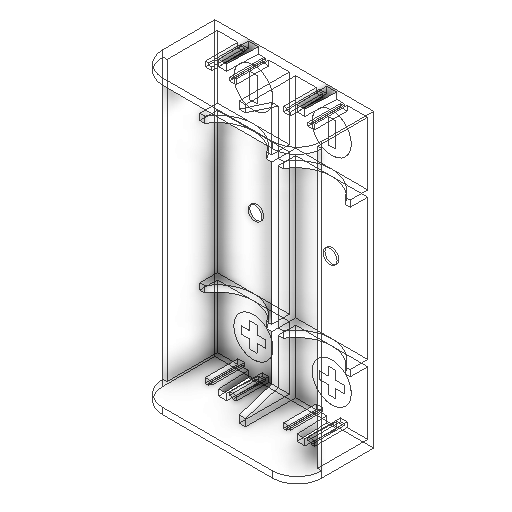
# Autodesk Inventor part: Holder_21700_Dual
Saved by Autodesk Inventor 2025.2 (Build 292293000, 293)
## iProperties
Created: 2025-03-09
Part Number: Holder_21700_Dual
Material: Generic
Document SubType Name: Modeling
Designer: ahorat
Density: 1 g/cm^3
Appearance: Default
Author: ahorat
Autodesk Inventor part; units mm, degrees
ref_plane "YZ Plane" through (0, 0, 0) normal (1, 0, 0) x (0, 1, 0)
ref_plane "XZ Plane" through (0, 0, 0) normal (0, 1, 0) x (-1, 0, 0)
sketch "Sketch1" plane through (0, 0, 0) normal (0, 1, 0) x (-1, 0, 0)
  line L0 (-22.6, 0) -> (22.6, 0)
  line L1 (22.6, 0) -> (22.6, 14.8)
  line L2 (15.6, 21.8) -> (-15.6, 21.8)
  line L3 (-22.6, 14.8) -> (-22.6, 0)
  arc A0 (-15.6, 21.8) -> (-22.6, 14.8) centre (-15.6, 14.8) ccw
  arc A1 (22.6, 14.8) -> (15.6, 21.8) centre (15.6, 14.8) ccw
  point P0 (0, 0)
  point P1 (22.6, 21.8)
  point P2 (0, 0)
  dimension "d0" = 21.8
  dimension "d1" = 45.2
  dimension "d2" = 7
  constraints: 8 end point, 4 point on circle, 4 tangent, 2 centre point, 2 parallel, 2 point on line, 1 coincident, 1 equal radius, 1 horizontal, 1 midpoint, 1 perpendicular
  measures "d0" distance of L0.end point (22.6, 21.8)
  measures "d1" distance between parallel lines of L3 L1
  measures "d2" radius of A0
extrude "Extrusion1" add sketch "Sketch1" along normal mid plane 83
sketch "Sketch2" plane through (-15.6, 41.5, 21.8) normal (0, 0, 1) x (1, 0, 0)
  line L0 (37, -81.2) -> (-5.8, -81.2)
  line L1 (-5.8, -81.2) -> (-5.8, -1.8)
  line L2 (-5.8, -1.8) -> (37, -1.8)
  line L3 (37, -1.8) -> (37, -81.2)
  line L4 (37, -81.2) -> (-5.8, -1.8) construction
  line L5 (-5.8, -81.2) -> (37, -1.8) construction
  line L6 (0, 0) -> (31.2, 0) projected
  line L7 (-7, -83) -> (-7, 0) projected
  point P0 (15.6, -41.5)
  dimension "d5" = 1.8
  dimension "d6" = 1.2
  constraints: 12 end point, 2 midpoint, 2 parallel, 1 horizontal, 1 perpendicular
  measures "d5" distance between parallel lines of L6 L2
  measures "d6" distance between parallel lines of L7 L1
extrude "Extrusion2" cut sketch "Sketch2" against normal blind 21.3
sketch "Sketch3" plane through (-15.6, -41.5, 21.8) normal (0, 0, 1) x (1, 0, 0)
  line L0 (65.6667, 1.8) -> (-34.4667, 1.8)
  line L1 (-34.4667, 1.8) -> (-34.4667, 81.2)
  line L2 (-34.4667, 81.2) -> (65.6667, 81.2)
  line L3 (65.6667, 81.2) -> (65.6667, 1.8)
  line L4 (65.6667, 1.8) -> (-34.4667, 81.2) construction
  line L5 (-34.4667, 1.8) -> (65.6667, 81.2) construction
  line L6 (0, 81.2) -> (31.2, 81.2) projected
  point P0 (15.6, 41.5)
  point P1 (15.6, 81.2)
  constraints: 12 end point, 4 midpoint, 2 parallel, 1 horizontal, 1 perpendicular
extrude "Extrusion3" cut sketch "Sketch3" against normal up to surface (7 mm away)
sketch "Sketch4" plane through (0, 0, 0) normal (1, 0, 0) x (0, 1, 0)
  line L0 (-39.7, 21.8) -> (-39.7, 14.8) projected
  line L1 (-39.7, 14.8) -> (-37.7, 14.8)
  line L2 (-39.7, 14.8) -> (39.7, 14.8) projected
  line L3 (-34.7, 5.5) -> (34.7, 5.5)
  line L4 (34.7, 5.5) -> (37.7, 14.8)
  line L5 (-34.7, 5.5) -> (-37.7, 14.8)
  line L6 (-39.7, 14.8) -> (-39.7, 0.5) projected
  line L7 (39.7, 0.5) -> (-39.7, 0.5) projected
  line L8 (39.7, 14.8) -> (39.7, 0.5) projected
  line L9 (0, 0) -> (0, 5.5) construction
  dimension "d11" = 2
  dimension "d12" = 5
  dimension "d13" = 5
  constraints: 10 end point, 2 point on line, 1 horizontal, 1 midpoint, 1 perpendicular, 1 other
  measures "d11" distance of L0.end L1.end
  measures "d12" distance between parallel lines of L7 L3
  measures "d13" distance from line of L3.start L6
extrude "Extrusion4" add sketch "Sketch4" along normal mid plane 1.8 contours L1 L5 L3 L4 L2 L8 L7 L6
ref_plane "Work Plane1" through (0, 0, 9.8) normal (0, 0, 1) x (1, 0, 0)
sketch "Sketch5" plane through (0, 0, 9.8) normal (0, 0, 1) x (1, 0, 0)
  line L0 (-0.9, -39.7) -> (-21.4, -39.7) projected
  line L1 (-15.55, -39.7) -> (-15.55, -38.3)
  line L2 (-15.55, -38.3) -> (-13.65, -38.3)
  line L3 (-13.65, -38.3) -> (-13.65, -39.2)
  line L4 (-13.65, -39.2) -> (-14.65, -39.2)
  line L5 (-14.65, -39.2) -> (-14.65, -39.7)
  line L6 (-7.65, -39.7) -> (-7.65, -39.2)
  line L7 (-7.65, -39.2) -> (-8.65, -39.2)
  line L8 (-8.65, -39.2) -> (-8.65, -38.3)
  line L9 (-8.65, -38.3) -> (-6.75, -38.3)
  line L10 (-6.75, -38.3) -> (-6.75, -39.7)
  line L11 (-13.65, -38.75) -> (-8.65, -38.75) construction
  line L12 (15.6, -39.7) -> (-15.6, -39.7) projected
  point P0 (0, 0)
  point P1 (-11.15, -38.75)
  point P2 (-11.15, -39.7)
  dimension "d17" = 0.9
  dimension "d18" = 0.9
  dimension "d19" = 7
  dimension "d20" = 0.5
  dimension "d21" = 5
  constraints: 22 end point, 8 point on line, 6 perpendicular, 4 midpoint, 2 collinear, 1 parallel, 1 vertical, 1 vertical alignment
  measures "d17" distance between parallel lines of L1 L5
  measures "d18" distance of L2.end L3.end
  measures "d19" distance between parallel lines of L5 L6
  measures "d20" distance of L4.end L5.end
  measures "d21" distance between parallel lines of L3 L8
extrude "Extrusion5" add sketch "Sketch5" against normal up to next
mirror "Mirror1" about plane through (0, 0, 0) normal (1, 0, 0) of "Extrusion5"
mirror "Mirror2" about plane through (0, 0, 0) normal (0, 1, 0) of "Extrusion5", "Mirror1"
sketch "Sketch6" plane through (0, 41.5, 0) normal (0, 1, 0) x (1, 0, 0)
  line L0 (14.65, -0.5) -> (7.65, -0.5) projected
  line L1 (12.26, -9.25) -> (10.04, -9.25)
  line L2 (10.04, -9.25) -> (9.71, -0.5)
  line L3 (12.26, -9.25) -> (12.59, -0.5)
  line L4 (12.425, -4.875) -> (9.875, -4.875) construction
  line L5 (0, 0) -> (0, -16.5721) construction
  line L6 (-12.26, -9.25) -> (-10.04, -9.25)
  line L7 (-10.04, -9.25) -> (-9.71, -0.5)
  line L8 (-12.26, -9.25) -> (-12.59, -0.5)
  line L9 (-12.425, -4.875) -> (-9.875, -4.875) construction
  line L10 (-9.71, -0.5) -> (-12.59, -0.5)
  line L11 (-7.65, -0.5) -> (-14.65, -0.5) projected
  point P0 (11.15, -9.25)
  point P1 (11.15, -0.5)
  point P2 (11.15, -4.875)
  point P3 (-11.15, -9.25)
  point P4 (-11.15, -0.5)
  point P5 (-11.15, -4.875)
  dimension "d24" = 2.22
  dimension "d25" = 2.88
  dimension "d26" = 8.75
  constraints: 20 end point, 10 symmetric about line, 5 midpoint, 2 point on line, 2 vertical alignment, 1 collinear, 1 horizontal, 1 vertical
  measures "d24" distance of L1.start L1.end
  measures "d25" distance of L3.end L2.end
  measures "d26" distance between parallel lines of L0 L1
extrude "Extrusion6" cut sketch "Sketch6" against normal through all
sketch "Sketch7" plane through (0, 0, 5.5) normal (0, 0, 1) x (1, 0, 0)
  line L0 (21.4, 39.7) -> (21.4, -39.7) projected
  line L1 (21.4, -21.8) -> (-21.4, -21.8)
  line L2 (-21.4, -21.8) -> (-21.4, -20)
  line L3 (-21.4, -20) -> (21.4, -20)
  line L4 (21.4, -20) -> (21.4, -21.8)
  line L5 (21.4, 20) -> (-21.4, 20)
  line L6 (-21.4, 20) -> (-21.4, 21.8)
  line L7 (-21.4, 21.8) -> (21.4, 21.8)
  line L8 (21.4, 21.8) -> (21.4, 20)
  line L9 (-21.4, 39.7) -> (-21.4, -39.7) projected
  line L10 (0, -20) -> (0, 20)
  point P0 (0, 0)
  point P1 (0, 0)
  dimension "d29" = 1.8
  dimension "d30" = 40
  constraints: 18 end point, 4 parallel, 4 point on line, 3 midpoint, 2 horizontal, 2 perpendicular, 1 coincident, 1 collinear
  measures "d29" distance of L1.end L2.end
  measures "d30" distance between parallel lines of L5 L3
extrude "Extrusion7" add sketch "Sketch7" against normal up to next contours L0 L5 L6 L7 | L0 L1 L2 L3
sketch "Sketch8" plane through (0.9, 21.8, 5.5) normal (0, 1, 0) x (1, 0, 0)
  circle A0 centre (10.25, -5.25) radius 10.25
  line L0 (8.81, 5) -> (11.69, 5) projected
  circle A1 centre (-12.05, -5.25) radius 10.25
  line L1 (-13.49, 5) -> (-10.61, 5) projected
  point P0 (-0.9, 5.5)
  point P1 (10.25, 5)
  point P2 (-12.05, 5)
  dimension "d33" = 20.5
  constraints: 2 centre point, 2 midpoint, 2 tangent, 2 vertical alignment, 1 equal radius
  measures "d33" diameter of A0
extrude "Extrusion8" cut sketch "Sketch8" against normal blind 50
sketch "Sketch9" plane through (-15.6, 41.5, 0.5) normal (0, 0, 1) x (1, 0, 0)
  line L0 (4.905, -41.5) -> (26.295, -41.5)
  line L1 (0, 0) -> (31.2, 0) projected
  line L2 (-7, -81.2) -> (-7, -1.8) projected
  point P0 (15.6, -41.5)
  point P1 (15.6, -41.5)
  point P2 (15.6, 0)
  point P3 (-7, -41.5)
  dimension "d43" = 21.39
  constraints: 3 midpoint, 2 end point, 1 horizontal, 1 horizontal alignment, 1 vertical alignment
  measures "d43" distance of L0.start L0.end
hole "Hole1" at (-10.695, 0, 0.5) at (10.695, 0, 0.5) direction (0, 0, -1) diameter 4 depth 1 tip angle 118
sketch "Sketch10" plane through (-15.6, 41.5, 0.5) normal (0, 0, 1) x (1, 0, 0)
  circle A0 centre (4.45, -72.25) radius 5.5798
  line L0 (-5.8, -81.2) -> (-5.8, -63.3) construction
  line L1 (3.412, -73.288) -> (0.95, -73.288)
  line L2 (0.95, -73.288) -> (0.95, -71.212)
  line L3 (0.95, -71.212) -> (3.412, -71.212)
  line L4 (3.412, -71.212) -> (3.412, -68.75)
  line L5 (3.412, -68.75) -> (5.488, -68.75)
  line L6 (5.488, -68.75) -> (5.488, -71.212)
  line L7 (5.488, -71.212) -> (7.95, -71.212)
  line L8 (7.95, -71.212) -> (7.95, -73.288)
  line L9 (7.95, -73.288) -> (5.488, -73.288)
  line L10 (5.488, -75.75) -> (3.412, -75.75)
  line L11 (3.412, -75.75) -> (3.412, -73.288)
  line L12 (5.488, -73.288) -> (5.488, -75.75)
  circle A1 centre (4.45, -10.75) radius 5.5798
  line L13 (-5.8, -19.7) -> (-5.8, -1.8) projected
  line L14 (5.488, -14.25) -> (3.412, -14.25)
  line L15 (3.412, -14.25) -> (3.412, -7.25)
  line L16 (3.412, -7.25) -> (5.488, -7.25)
  line L17 (5.488, -7.25) -> (5.488, -14.25)
  line L18 (5.488, -14.25) -> (3.412, -7.25) construction
  line L19 (3.412, -14.25) -> (5.488, -7.25) construction
  point P0 (15.6, -41.5)
  point P1 (4.45, -63.3)
  point P2 (-5.8, -72.25)
  point P3 (4.45, -68.75)
  point P4 (0.95, -72.25)
  point P5 (-5.8, -10.75)
  point P6 (4.45, -19.7)
  dimension "d44" = 7
  dimension "d45" = 7
  constraints: 36 end point, 9 point on line, 7 perpendicular, 6 midpoint, 5 equal length, 3 horizontal alignment, 3 parallel, 3 vertical alignment, 2 centre point, 2 horizontal, 1 equal radius, 1 vertical
  measures "d44" distance of L14.end L15.end
  measures "d45" distance between parallel lines of L10 L5
extrude "Extrusion9" cut sketch "Sketch10" against normal blind 0.01
mirror "Mirror3" about plane through (0, 0, 0) normal (1, 0, 0) of "Extrusion9"
body "Solid1"
